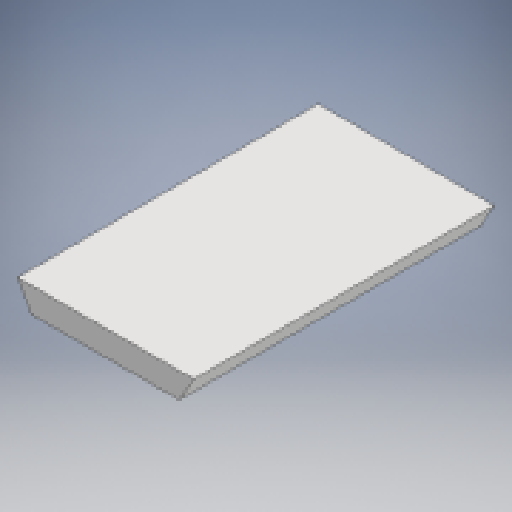
# Autodesk Inventor part: Part6
Saved by Autodesk Inventor 2025.2 (Build 292293000, 293)
## iProperties
Created: 2025-02-14
Part Number: Part6
Material: Generic
Document SubType Name: Modeling
Designer: Alex
Density: 1 g/cm^3
Appearance: Default
Author: Alex
Autodesk Inventor part; units mm, degrees
ref_plane "YZ Plane" through (0, 0, 0) normal (1, 0, 0) x (0, 1, 0)
ref_plane "XZ Plane" through (0, 0, 0) normal (0, 1, 0) x (-1, 0, 0)
ref_plane "XY Plane" through (0, 0, 0) normal (0, 0, 1) x (1, 0, 0)
sketch "Sketch1" plane through (0, 0, 0) normal (0, 0, 1) x (1, 0, 0)
  line L0 (39.4171, 0) -> (37.6851, -3) projected
  line L1 (6.8453, -3) -> (5.1132, 0) projected
  line L2 (5.1132, 0) -> (39.4171, 0) projected
  line L3 (36.3139, -4.875) -> (38.9841, -0.25)
  line L4 (38.9841, -0.25) -> (5.5463, -0.25)
  line L5 (5.5463, -0.25) -> (8.2165, -4.875)
  line L6 (36.3139, -4.875) -> (36.2417, -5)
  line L7 (8.2165, -4.875) -> (8.2887, -5)
  line L8 (8.2887, -5) -> (36.2417, -5)
  point P0 (0, 0)
  dimension "d0" = 0.25
  dimension "d1" = 4.75
  constraints: 12 end point, 2 collinear, 1 horizontal, 2 other
  measures "d0" distance between parallel lines of L2 L4
  measures "d1" distance between parallel lines of L4 L8
extrude "Extrusion1" add sketch "Sketch1" against normal blind 57
sketch "Sketch2" plane through (5.5463, -0.25, 0) normal (0, 1, 0) x (1, 0, 0)
  circle A0 centre (16.7189, 3) radius 0.922 projected
  point P0 (-5.5463, 0)
ref_plane "Work Plane1" through (22.2652, -0.25, -3) normal (0, 0, 1) x (1, 0, 0)
sketch "Sketch3" plane through (22.2652, -0.25, -3) normal (0, 0, 1) x (1, 0, 0)
  line L0 (-16.7189, 0) -> (16.7189, 0) construction
  line L1 (0, 0) -> (0, 0.85) construction
  arc A0 (0.7775, 0.3597) -> (-0.7775, 0.3597) centre (0, 0.1429) ccw construction
  arc A1 (0, 0.85) -> (-0.75, 0) centre (0, 0.0941) ccw
  line L2 (-0.75, 0) -> (0, 0)
  line L3 (0, 0) -> (0, 0.85)
  point P0 (-22.2652, 0.25)
  dimension "d4" = 0.85
  dimension "d5" = 0.75
  constraints: 6 end point, 4 point on circle, 2 centre point, 2 collinear, 1 line through centre, 1 midpoint, 1 point on line, 1 vertical, 4 other
  measures "d4" distance of L1.start L1.end
  measures "d5" distance of L2.start L1.start
revolve "Revolution1" add sketch "Sketch3" angle 360 about axis through (22.2652, -0.25, -3) along (0, 1, 0)
fillet "Fillet1" radius 0.18 1 edges at (23.0152, -0.25, -3)
fillet "Fillet2" radius 2 1 edges at (22.2652, -5, 0)
body "Solid1"
